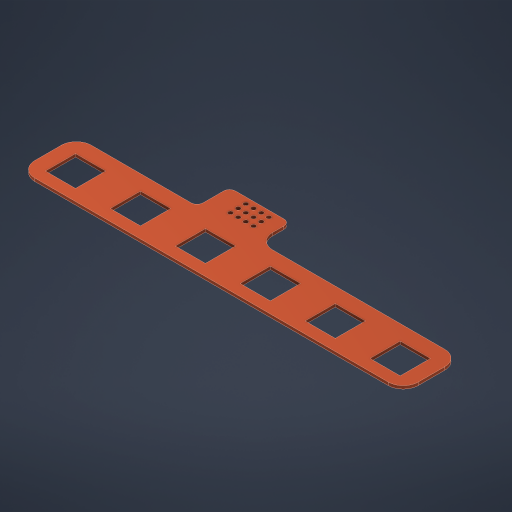
# Autodesk Inventor part: bat_contacts_v2_plate_contact
Saved by Autodesk Inventor 2024.3 (Build 283343010, 343A)
## iProperties
Created: 2025-05-07
Part Number: bat_contacts_v2_plate_contact
Material: Kupfer
Document SubType Name: Modellieren
Designer: David
Density: 8.94 g/cm^3
Appearance: Kupfer - satiniert
Sheet Metal Rule: Standard_mm
Author: David
Autodesk Inventor part; units mm, degrees
ref_plane "YZ Plane" through (0, 0, 0) normal (1, 0, 0) x (0, 1, 0)
ref_plane "XZ Plane" through (0, 0, 0) normal (0, 1, 0) x (-1, 0, 0)
ref_plane "XY Plane" through (0, 0, 0) normal (0, 0, 1) x (1, 0, 0)
sketch "Skizze1" plane through (0, 0, 0) normal (0, 0, 1) x (1, 0, 0)
  line L0 (0, 0) -> (127, 0)
  line L1 (127, 0) -> (127, 37.5)
  line L2 (127, 37.5) -> (0, 37.5)
  line L3 (0, 37.5) -> (0, 0)
  line L4 (4.75, 3.75) -> (14.75, 3.75)
  line L5 (14.75, 3.75) -> (14.75, 13.75)
  line L6 (14.75, 13.75) -> (4.75, 13.75)
  line L7 (4.75, 13.75) -> (4.75, 3.75)
  line L8 (4.75, 33.75) -> (4.75, 23.75)
  line L9 (14.75, 33.75) -> (4.75, 33.75)
  line L10 (14.75, 23.75) -> (14.75, 33.75)
  line L11 (4.75, 23.75) -> (14.75, 23.75)
  line L12 (26.25, 13.75) -> (26.25, 3.75)
  line L13 (36.25, 13.75) -> (26.25, 13.75)
  line L14 (36.25, 3.75) -> (36.25, 13.75)
  line L15 (26.25, 3.75) -> (36.25, 3.75)
  line L16 (26.25, 33.75) -> (26.25, 23.75)
  line L17 (36.25, 33.75) -> (26.25, 33.75)
  line L18 (36.25, 23.75) -> (36.25, 33.75)
  line L19 (26.25, 23.75) -> (36.25, 23.75)
  line L20 (47.75, 13.75) -> (47.75, 3.75)
  line L21 (57.75, 13.75) -> (47.75, 13.75)
  line L22 (57.75, 3.75) -> (57.75, 13.75)
  line L23 (47.75, 3.75) -> (57.75, 3.75)
  line L24 (47.75, 33.75) -> (47.75, 23.75)
  line L25 (57.75, 33.75) -> (47.75, 33.75)
  line L26 (57.75, 23.75) -> (57.75, 33.75)
  line L27 (47.75, 23.75) -> (57.75, 23.75)
  line L28 (69.25, 13.75) -> (69.25, 3.75)
  line L29 (79.25, 13.75) -> (69.25, 13.75)
  line L30 (79.25, 3.75) -> (79.25, 13.75)
  line L31 (69.25, 3.75) -> (79.25, 3.75)
  line L32 (69.25, 33.75) -> (69.25, 23.75)
  line L33 (79.25, 33.75) -> (69.25, 33.75)
  line L34 (79.25, 23.75) -> (79.25, 33.75)
  line L35 (69.25, 23.75) -> (79.25, 23.75)
  line L36 (90.75, 13.75) -> (90.75, 3.75)
  line L37 (100.75, 13.75) -> (90.75, 13.75)
  line L38 (100.75, 3.75) -> (100.75, 13.75)
  line L39 (90.75, 3.75) -> (100.75, 3.75)
  line L40 (90.75, 33.75) -> (90.75, 23.75)
  line L41 (100.75, 33.75) -> (90.75, 33.75)
  line L42 (100.75, 23.75) -> (100.75, 33.75)
  line L43 (90.75, 23.75) -> (100.75, 23.75)
  line L44 (112.25, 13.75) -> (112.25, 3.75)
  line L45 (122.25, 13.75) -> (112.25, 13.75)
  line L46 (122.25, 3.75) -> (122.25, 13.75)
  line L47 (112.25, 3.75) -> (122.25, 3.75)
  line L48 (112.25, 33.75) -> (112.25, 23.75)
  line L49 (122.25, 33.75) -> (112.25, 33.75)
  line L50 (122.25, 23.75) -> (122.25, 33.75)
  line L51 (112.25, 23.75) -> (122.25, 23.75)
  line L52 (0, 18.75) -> (40, 18.75)
  line L53 (40, 18.75) -> (40, 29.5)
  line L54 (40, 29.5) -> (60, 29.5)
  line L55 (60, 29.5) -> (60, 23.75)
  arc A0 (60, 23.75) -> (65, 18.75) centre (65, 23.75) ccw
  line L56 (65, 18.75) -> (127, 18.75)
  point P0 (63.5, 37.5)
  point P1 (42, 18.75)
  point P2 (85, 18.75)
  point P3 (63.5, 0)
  point P4 (55, 27.5)
  point P5 (52.46, 27.5)
  point P6 (49.92, 27.5)
  point P7 (47.38, 27.5)
  point P8 (55, 24.96)
  point P9 (52.46, 24.96)
  point P10 (49.92, 24.96)
  point P11 (47.38, 24.96)
  point P12 (55, 22.42)
  point P13 (52.46, 22.42)
  point P14 (49.92, 22.42)
  point P15 (47.38, 22.42)
  dimension "d0" = 127
  dimension "d1" = 37.5
  dimension "d2" = 10
  dimension "d3" = 10
  dimension "d6" = 20
  dimension "d9" = 21.5
  dimension "d12" = 5
  dimension "d13" = 5.75
  dimension "d17" = 43
  dimension "d18" = 21.5
  dimension "d19" = 29.5
  dimension "d20" = 60
  dimension "d21" = 5
  dimension "d22" = 20
  dimension "d23" = 2
  dimension "d24" = 5
  dimension "d36" = 2.54
  dimension "d39" = 2.54
  constraints: 114 end point, 5 horizontal, 5 perpendicular, 4 midpoint, 4 parallel, 2 horizontal alignment, 2 point on circle, 2 tangent, 2 vertical, 1 centre point, 1 point on line, 99 other
  measures "d0" distance of L1.end L2.end
  measures "d1" distance of L2.end L0.start
  measures "d2" distance of L6.end L4.start
  measures "d3" distance of L4.start L4.end
  measures "d6" distance of L6.end L8.start
  measures "d9" distance of L6.end L12.start
  measures "d12" distance from line of L52.start L11
  measures "d13" distance from line of point (63.5, 37.5) L26
  measures "d17" distance of point (85, 18.75) point (42, 18.75)
  measures "d18" horizontal distance of point (63.5, 0) point (42, 18.75)
  measures "d19" distance between parallel lines of L0 L54
  measures "d20" distance between parallel lines of L3 L55
  measures "d21" radius of A0
  measures "d22" distance of L53.end L54.end
  measures "d23" distance from line of point (55, 27.5) L54
  measures "d24" distance from line of L55 point (55, 27.5)
  measures "d36" distance of point (55, 27.5) point (52.46, 27.5)
  measures "d39" distance of point (55, 27.5) point (55, 24.96)
extrude "Extrusion1" add sketch "Skizze1" along normal blind 1 contours L3 L52 L53 L54 L24 L27 L26 L55 A0 L56 L1 L0 | L54 L26 L27 L24
fillet "Rundung1" radius 5 2 edges at (127, 0, 0.5) (0, 0, 0.5)
hole "Bohrung1" at (55, 27.5, 0) at (55, 24.96, 0) at (52.46, 24.96, 0) at (49.92, 24.96, 0) at (49.92, 27.5, 0) at (52.46, 27.5, 0) at (55, 22.42, 0) at (52.46, 22.42, 0) at (49.92, 22.42, 0) at (47.38, 22.42, 0) at (47.38, 24.96, 0) at (47.38, 27.5, 0) direction (0, 0, 1) diameter 1.475 end through all
fillet "Rundung2" radius 2 3 edges at (60, 29.5, 0.5) (40, 18.75, 0.5) (40, 29.5, 0.5)
fillet "Rundung3" radius 5 2 edges at (0, 18.75, 0.5) (127, 18.75, 0.5)
sketch "Skizze2" plane through (0, 0, 1) normal (0, 0, 1) x (1, 0, 0)
  arc A0 (0, 5) -> (5, 0) centre (5, 5) ccw projected
  line L0 (5, 0) -> (122, 0) projected
  arc A1 (122, 0) -> (127, 5) centre (122, 5) ccw projected
  line L1 (127, 5) -> (127, 13.75) projected
  line L2 (0, 13.75) -> (0, 5) projected
  line L3 (112.25, 13.75) -> (122.25, 13.75) projected
  line L4 (122.25, 13.75) -> (122.25, 3.75) projected
  line L5 (122.25, 3.75) -> (112.25, 3.75) projected
  line L6 (112.25, 3.75) -> (112.25, 13.75) projected
  line L7 (90.75, 13.75) -> (100.75, 13.75) projected
  line L8 (100.75, 13.75) -> (100.75, 3.75) projected
  line L9 (100.75, 3.75) -> (90.75, 3.75) projected
  line L10 (90.75, 3.75) -> (90.75, 13.75) projected
  line L11 (69.25, 13.75) -> (79.25, 13.75) projected
  line L12 (79.25, 13.75) -> (79.25, 3.75) projected
  line L13 (79.25, 3.75) -> (69.25, 3.75) projected
  line L14 (69.25, 3.75) -> (69.25, 13.75) projected
  line L15 (47.75, 13.75) -> (57.75, 13.75) projected
  line L16 (57.75, 13.75) -> (57.75, 3.75) projected
  line L17 (57.75, 3.75) -> (47.75, 3.75) projected
  line L18 (47.75, 3.75) -> (47.75, 13.75) projected
  line L19 (26.25, 13.75) -> (36.25, 13.75) projected
  line L20 (36.25, 13.75) -> (36.25, 3.75) projected
  line L21 (36.25, 3.75) -> (26.25, 3.75) projected
  line L22 (26.25, 3.75) -> (26.25, 13.75) projected
  line L23 (4.75, 3.75) -> (4.75, 13.75) projected
  line L24 (4.75, 13.75) -> (14.75, 13.75) projected
  line L25 (14.75, 13.75) -> (14.75, 3.75) projected
  line L26 (14.75, 3.75) -> (4.75, 3.75) projected
  line L27 (122, 18.75) -> (65, 18.75) projected
  arc A2 (60, 23.75) -> (65, 18.75) centre (65, 23.75) ccw projected
  line L28 (60, 23.75) -> (60, 27.5) projected
  line L29 (58, 29.5) -> (42, 29.5) projected
  line L30 (40, 27.5) -> (40, 20.75) projected
  line L31 (38, 18.75) -> (5, 18.75) projected
  arc A3 (127, 13.75) -> (122, 18.75) centre (122, 13.75) ccw projected
  arc A4 (60, 27.5) -> (58, 29.5) centre (58, 27.5) ccw projected
  arc A5 (42, 29.5) -> (40, 27.5) centre (42, 27.5) ccw projected
  arc A6 (38, 18.75) -> (40, 20.75) centre (38, 20.75) ccw projected
  arc A7 (5, 18.75) -> (0, 13.75) centre (5, 13.75) ccw projected
  circle A8 centre (55, 27.5) radius 0.7375 projected
  point P0 (0, 0)
equation "\"d12\" = 0.5 * d2"
equation "\"d13\" = -0.5 * d3 + 0.5 * d9"
equation "\"d17\" = 2 * d9"
equation "\"d18\" = 0.5 * d17"
equation "\"Biegeradius\" = Stärke"
equation "\"BreiteBiegungsfreistellung\" = Stärke"
equation "\"TiefeBiegungsfreistellung\" = 0.5 * Stärke"
equation "\"GrößeEckenfreistellung\" = 4 * Stärke"
equation "\"MinimalRest\" = 2 * Stärke"
equation "\"Übergangsradius\" = Biegeradius"
equation "\"JacobiRadiusGröße\" = Biegeradius"
equation "\"Abstandsgröße\" = Stärke"
equation "\"Stärke\" = 0.5"
